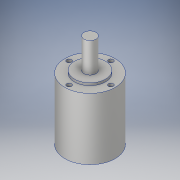
# Autodesk Inventor part: 27-1 Gearbox
Saved by Autodesk Inventor 2019.4 (Build 234330000, 330)
## iProperties
Created: 2019-11-30
Part Number: 27-1 Gearbox
Material: Aluminum 6061
Document SubType Name: Modeling
Designer: admin
Density: 4.97302 g/cm^3
Appearance: Aluminum - Flat
Mass: 370 g
Surface Area: 107.926 cm^2
Volume: 74.4014 cm^3
Author: admin
Autodesk Inventor part; units mm, degrees
ref_plane "YZ Plane" through (0, 0, 0) normal (1, 0, 0) x (0, 1, 0)
ref_plane "XZ Plane" through (0, 0, 0) normal (0, 1, 0) x (-1, 0, 0)
ref_plane "XY Plane" through (0, 0, 0) normal (0, 0, 1) x (1, 0, 0)
sketch "Sketch1" plane through (0, 0, 0) normal (0, 1, 0) x (-1, 0, 0)
  circle A0 centre (0, 0) radius 21
  dimension "d0" = 42
  constraints: 1 centre point, 1 coincident
  measures "d0" diameter of A0
extrude "Extrusion1" add sketch "Sketch1" along normal blind 51.7
sketch "Sketch2" plane through (0, 51.7, 0) normal (0, 1, 0) x (1, 0, 0)
  circle A0 centre (0, 0) radius 13
  dimension "d3" = 26
  constraints: 1 centre point, 1 coincident
  measures "d3" diameter of A0
extrude "Extrusion2" add sketch "Sketch2" along normal blind 2
sketch "Sketch3" plane through (0, 53.7, 0) normal (0, 1, 0) x (1, 0, 0)
  circle A0 centre (0, 0) radius 5
  dimension "d6" = 10
  constraints: 1 centre point, 1 coincident
  measures "d6" diameter of A0
extrude "Extrusion3" add sketch "Sketch3" along normal blind 25
sketch "Sketch4" plane through (0, 51.7, 0) normal (0, 1, 0) x (1, 0, 0)
  circle A0 centre (0, -17.5) radius 2
  line L0 (0, -17.5) -> (0, 0) construction
  circle A1 centre (17.5, 0) radius 2
  circle A2 centre (0, 17.5) radius 2
  circle A3 centre (-17.5, 0) radius 2
  dimension "d9" = 4
  dimension "d10" = 17.5
  dimension "d13" = 360
  constraints: 4 centre point, 2 end point, 1 vertical, 9 other
  measures "d9" diameter of A0
  measures "d10" distance of L0.start L0.end
extrude "Extrusion4" cut sketch "Sketch4" against normal blind 5
body "Solid1"
